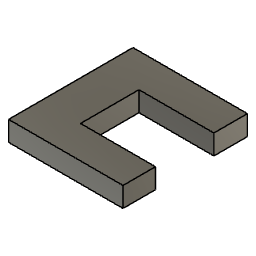
C letter v1 (Autodesk Fusion 360 design; units mm, degrees)
Autodesk Fusion 360 part; units mm, degrees
sketch "Sketch1" plane through (0, 0, 0) normal (0, 0, 1) x (1, 0, 0)
  line L0 (0.0247, 50.0428) -> (30.0247, 50.0428)
  line L1 (30.0247, 50.0428) -> (30.0247, 25.0428)
  line L2 (30.0247, 25.0428) -> (0.0247, 25.0428)
  line L3 (0.0247, 25.0428) -> (0.0247, 50.0428)
  dimension "d3" = 30
  dimension "d4" = 25
  constraint horizontal L0
  constraint vertical L1
  constraint horizontal L2
  constraint vertical L3
  measures "d3" distance of L0.start L0.end
  measures "d4" distance of L0.start L2.end
extrude "Extrude1" add sketch "Sketch1" along normal blind 4
sketch "Sketch2" plane through (0, 0, 0) normal (0, 0, 1) x (1, 0, 0)
  line L0 (7.9626, 43.3083) -> (30.0026, 43.3083)
  line L1 (30.0026, 43.3083) -> (30.0026, 31.5625)
  line L2 (30.0026, 31.5625) -> (7.9626, 31.5625)
  line L3 (7.9626, 31.5625) -> (7.9626, 43.3083)
  constraint horizontal L0
  constraint vertical L1
  constraint horizontal L2
  constraint vertical L3
extrude "Extrude2" cut sketch "Sketch2" along normal blind 4
extrude "Extrude3" cut 1 faces at (30.0247, 41.7095, 1.3333) along direction (-1, 0, 0) blind 7
